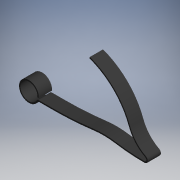
# Autodesk Inventor part: scissor_spring
Saved by Autodesk Inventor 2019 (Build 230136000, 136)
## iProperties
Shininess: 0.0
Length Units: 11269
Angle Units: 11279
Time Units: 11290
Mass Units: 11283
Length Display Precision: 3
Angle Display Precision: 2
Compacted: True
Company: Autodesk
Created: 2000-05-30
Part Number: scissor_spring
Document SubType Name: Modeling
Designer: Autodesk, Inc.
Mass: 0.0153082 g
Surface Area: 1.69192 cm^2
Volume: 0.0153082 cm^3
Density: 1 g/cm^3
Material: Generic
Appearance: Rubber-Black
Density: 0.0
Volumn: 0.0
Area: 0.0
PropertySet Name: Model Information
Control State: 0
Master: False
Checked Out: False
Author: Autodesk, Inc.
Autodesk Inventor part; units mm, degrees
ref_plane "YZ Plane" through (0, 0, 0) normal (1, 0, 0) x (0, 1, 0)
ref_plane "XZ Plane" through (0, 0, 0) normal (0, 1, 0) x (-1, 0, 0)
ref_plane "XY Plane" through (0, 0, 0) normal (0, 0, 1) x (1, 0, 0)
sketch "Sketch1" plane through (0, 0, 0) normal (0, 0, 1) x (1, 0, 0)
  arc A0 (-2.8862, -1.2447) -> (-2.6561, -0.3007) centre (-2.8862, -0.7447) ccw
  arc A1 (-7.2602, -0.8985) -> (-2.8862, -1.2447) centre (-2.8862, 26.566) ccw
  arc A2 (-5.0488, 2.4151) -> (-2.6561, -0.3007) centre (-0.3551, 4.1384) ccw
  arc A3 (-5.0488, 2.4151) -> (-11.1621, 8.4942) centre (-14.6238, -1.1004) ccw
  arc A4 (-16.9335, -1.2455) -> (-10.6071, -0.846) centre (-16.9124, 48.7131) ccw
  arc A5 (-7.2602, -0.8985) -> (-10.6071, -0.846) centre (-9.1171, -12.5575) ccw
  arc A6 (-16.9335, -1.0455) -> (-10.6324, -0.6476) centre (-16.9124, 48.7131) ccw
  arc A7 (-7.2288, -0.701) -> (-10.6324, -0.6476) centre (-9.1171, -12.5575) ccw
  arc A8 (-7.2288, -0.701) -> (-2.8862, -1.0447) centre (-2.8862, 26.566) ccw
  arc A9 (-2.8862, -1.0447) -> (-2.7481, -0.4783) centre (-2.8862, -0.7447) ccw
  arc A10 (-5.2365, 2.3461) -> (-2.7481, -0.4783) centre (-0.3551, 4.1384) ccw
  arc A11 (-5.2365, 2.3461) -> (-11.23, 8.3061) centre (-14.6238, -1.1004) ccw
  line L0 (-11.1621, 8.4942) -> (-11.23, 8.3061)
  line L1 (-5.2365, 2.3461) -> (-5.0488, 2.4151) construction
  line L2 (-2.7481, -0.4783) -> (-2.6561, -0.3007) construction
  line L3 (-5.0488, 2.4151) -> (-0.3551, 4.1384) construction
  line L4 (-0.3551, 4.1384) -> (-2.6561, -0.3007) construction
  line L5 (-11.23, 8.3061) -> (-14.6238, -1.1004) construction
  arc A12 (-18.8918, -0.7763) -> (-19.0627, -1.3505) centre (-20.3859, -0.644) ccw projected
  arc A13 (-18.8862, -1.2447) -> (-19.0627, -1.3505) centre (-18.8862, -1.4447) ccw projected
  arc A14 (-19.0927, -0.7763) -> (-19.2391, -1.2563) centre (-20.3859, -0.644) ccw
  arc A15 (-18.8861, -1.0447) -> (-19.2391, -1.2563) centre (-18.8862, -1.4447) ccw
  line L6 (-18.8862, -1.2447) -> (-16.9335, -1.2455)
  line L7 (-18.8861, -1.0447) -> (-16.9335, -1.0455)
  line L8 (-18.8862, -1.2447) -> (-2.8862, -1.2447) construction
  line L9 (-19.0927, -0.7763) -> (-18.8918, -0.7763)
  point P0 (-18.8374, -1.1048)
  dimension "d25" = 50
  dimension "d26" = 42.44
  dimension "d27" = 10
  dimension "d28" = 5
  dimension "d34" = 0.5
  dimension "d35" = 1.3
  dimension "d36" = 16
  constraints: 28 point on circle, 20 end point, 15 tangent, 14 centre point, 3 collinear, 2 parallel, 1 horizontal, 2 other
  measures "d25" angle of L3 L5
  measures "d26" angle of L4 L3
  measures "d27" radius of A11
  measures "d28" radius of A2
  measures "d34" radius of A0
  measures "d35" radius of A14
  measures "d36" distance of L6.start L8.end
extrude "Extrusion2" add sketch "Sketch1" against normal blind 2
body "Solid1"
